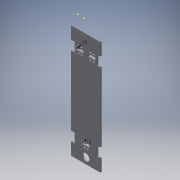
# Autodesk Inventor part: XCartFloor
Saved by Autodesk Inventor 2019 (Build 230136000, 136)
## iProperties
Created: 2019-08-19
Part Number: XCartFloor
Material: Generic
Document SubType Name: Modeling
Designer: Bruno
Density: 1 g/cm^3
Appearance: Default
Author: Bruno
Autodesk Inventor part; units mm, degrees
ref_plane "YZ Plane" through (0, 0, 0) normal (1, 0, 0) x (0, 1, 0)
ref_plane "XZ Plane" through (0, 0, 0) normal (0, 1, 0) x (-1, 0, 0)
ref_plane "XY Plane" through (0, 0, 0) normal (0, 0, 1) x (1, 0, 0)
sketch "Sketch1" plane through (0, 0, 0) normal (0, 0, 1) x (1, 0, 0)
  line L0 (100.0979, -38.5222) -> (0.0979, -38.5222)
  line L1 (0.0979, -426.5222) -> (100.0979, -426.5222)
  line L2 (82.7645, -93.1222) -> (58.7645, -93.1222)
  line L3 (58.7645, -93.1222) -> (58.7645, -101.9222)
  line L4 (58.7645, -101.9222) -> (82.7645, -101.9222)
  line L5 (82.7645, -101.9222) -> (82.7645, -93.1222)
  line L6 (41.4312, -93.1222) -> (17.4312, -93.1222)
  line L7 (17.4312, -93.1222) -> (17.4312, -101.9222)
  line L8 (17.4312, -101.9222) -> (41.4312, -101.9222)
  line L9 (41.4312, -101.9222) -> (41.4312, -93.1222)
  line L10 (38.0979, -363.1222) -> (62.0979, -363.1222)
  line L11 (62.0979, -363.1222) -> (62.0979, -371.9222)
  line L12 (62.0979, -371.9222) -> (38.0979, -371.9222)
  line L13 (38.0979, -371.9222) -> (38.0979, -363.1222)
  line L14 (173.8639, -93.5222) -> (-221.1361, -93.5222)
  line L15 (173.8639, -101.5222) -> (-221.1361, -101.5222)
  line L16 (173.8639, -371.5222) -> (-221.1361, -371.5222)
  line L17 (173.8639, -363.5222) -> (-221.1361, -363.5222)
  line L18 (34.8712, -93.1222) -> (34.8712, -93.5222) construction
  line L19 (34.8712, -101.5222) -> (34.8712, -101.9222) construction
  line L20 (58.7645, -93.1222) -> (41.4312, -93.1222) construction
  line L21 (10.9151, -363.1222) -> (10.9151, -363.5222) construction
  line L22 (10.9151, -371.5222) -> (10.9151, -371.9222) construction
  line L23 (38.0979, -363.1222) -> (12.0979, -363.1222) construction
  line L24 (62.0979, -363.1222) -> (88.0979, -363.1222) construction
  line L25 (0, 0) -> (0, -9.7735) construction
  circle A0 centre (65.5981, -390.5222) radius 1.625
  circle A1 centre (65.5981, -421.5222) radius 1.625
  circle A2 centre (34.5981, -421.5222) radius 1.625
  circle A3 centre (34.5981, -390.5222) radius 1.625
  line L26 (65.5981, -390.5222) -> (34.5981, -390.5222) construction
  line L27 (34.5981, -390.5222) -> (34.5981, -421.5222) construction
  line L28 (34.5981, -421.5222) -> (65.5981, -421.5222) construction
  line L29 (65.5981, -421.5222) -> (65.5981, -390.5222) construction
  line L30 (34.5981, -390.5222) -> (0.0979, -390.3972) construction
  line L31 (65.5981, -390.5222) -> (100.0979, -390.7595) construction
  circle A4 centre (50.0981, -406.0222) radius 12.5
  line L32 (50.0981, -390.5222) -> (50.0981, -406.0222) construction
  line L33 (50.0981, -406.0222) -> (65.5981, -406.0222) construction
  line L34 (72.2645, -84.1222) -> (80.2645, -84.1222)
  line L35 (80.2645, -84.1222) -> (80.2645, -88.1222)
  line L36 (80.2645, -88.1222) -> (72.2645, -88.1222)
  line L37 (72.2645, -88.1222) -> (72.2645, -84.1222)
  line L38 (80.2645, -88.1222) -> (82.7645, -88.1222) construction
  line L39 (82.7645, -88.1222) -> (82.7645, -93.1222) construction
  line L40 (69.2645, -84.1222) -> (61.2645, -84.1222)
  line L41 (61.2645, -84.1222) -> (61.2645, -88.1222)
  line L42 (61.2645, -88.1222) -> (69.2645, -88.1222)
  line L43 (69.2645, -88.1222) -> (69.2645, -84.1222)
  line L44 (58.7645, -93.1222) -> (58.7645, -88.1222) construction
  line L45 (58.7645, -88.1222) -> (61.2645, -88.1222) construction
  line L46 (72.2645, -106.9222) -> (80.2645, -106.9222)
  line L47 (80.2645, -106.9222) -> (80.2645, -110.9222)
  line L48 (80.2645, -110.9222) -> (72.2645, -110.9222)
  line L49 (72.2645, -110.9222) -> (72.2645, -106.9222)
  line L50 (80.2645, -106.9222) -> (80.2645, -101.9222) construction
  line L51 (69.2645, -106.9222) -> (61.2645, -106.9222)
  line L52 (61.2645, -106.9222) -> (61.2645, -110.9222)
  line L53 (61.2645, -110.9222) -> (69.2645, -110.9222)
  line L54 (69.2645, -110.9222) -> (69.2645, -106.9222)
  line L55 (38.9312, -84.1222) -> (30.9312, -84.1222)
  line L56 (30.9312, -84.1222) -> (30.9312, -88.1222)
  line L57 (30.9312, -88.1222) -> (38.9312, -88.1222)
  line L58 (38.9312, -88.1222) -> (38.9312, -84.1222)
  line L59 (27.9312, -84.1222) -> (19.9312, -84.1222)
  line L60 (19.9312, -84.1222) -> (19.9312, -88.1222)
  line L61 (19.9312, -88.1222) -> (27.9312, -88.1222)
  line L62 (27.9312, -88.1222) -> (27.9312, -84.1222)
  line L63 (30.9312, -106.9222) -> (38.9312, -106.9222)
  line L64 (38.9312, -106.9222) -> (38.9312, -110.9222)
  line L65 (38.9312, -110.9222) -> (30.9312, -110.9222)
  line L66 (30.9312, -110.9222) -> (30.9312, -106.9222)
  line L67 (27.9312, -106.9222) -> (19.9312, -106.9222)
  line L68 (19.9312, -106.9222) -> (19.9312, -110.9222)
  line L69 (19.9312, -110.9222) -> (27.9312, -110.9222)
  line L70 (27.9312, -110.9222) -> (27.9312, -106.9222)
  line L71 (41.4312, -93.1222) -> (41.4312, -88.1222) construction
  line L72 (41.4312, -88.1222) -> (38.9312, -88.1222) construction
  line L73 (17.4312, -93.1222) -> (17.4312, -88.1222) construction
  line L74 (17.4312, -88.1222) -> (19.9312, -88.1222) construction
  line L75 (51.5979, -354.1222) -> (59.5979, -354.1222)
  line L76 (59.5979, -354.1222) -> (59.5979, -358.1222)
  line L77 (59.5979, -358.1222) -> (51.5979, -358.1222)
  line L78 (51.5979, -358.1222) -> (51.5979, -354.1222)
  line L79 (48.5979, -354.1222) -> (40.5979, -354.1222)
  line L80 (40.5979, -354.1222) -> (40.5979, -358.1222)
  line L81 (40.5979, -358.1222) -> (48.5979, -358.1222)
  line L82 (48.5979, -358.1222) -> (48.5979, -354.1222)
  line L83 (51.5979, -376.9222) -> (59.5979, -376.9222)
  line L84 (59.5979, -376.9222) -> (59.5979, -380.9222)
  line L85 (59.5979, -380.9222) -> (51.5979, -380.9222)
  line L86 (51.5979, -380.9222) -> (51.5979, -376.9222)
  line L87 (48.5979, -376.9222) -> (40.5979, -376.9222)
  line L88 (40.5979, -376.9222) -> (40.5979, -380.9222)
  line L89 (40.5979, -380.9222) -> (48.5979, -380.9222)
  line L90 (48.5979, -380.9222) -> (48.5979, -376.9222)
  line L91 (59.5979, -358.1222) -> (62.0979, -358.1222) construction
  line L92 (62.0979, -358.1222) -> (62.0979, -363.1222) construction
  line L93 (38.0979, -363.1222) -> (38.0979, -358.1222) construction
  line L94 (38.0979, -358.1222) -> (40.5979, -358.1222) construction
  line L95 (59.5979, -376.9222) -> (59.5979, -371.9222) construction
  circle A5 centre (73.5, -50.5222) radius 2.125
  circle A6 centre (26.5, -50.5222) radius 2.125
  line L96 (73.5, -50.5222) -> (100, -50.5222) construction
  line L97 (26.5, -50.5222) -> (0, -50.5222) construction
  line L98 (96.5, -57.5222) -> (88.5, -57.5222) projected
  line L99 (11.5, -57.5222) -> (3.5, -57.5222) projected
  line L100 (8, -43.5222) -> (8, -57.5222) projected
  line L101 (7, -57.5222) -> (7, -43.5222) projected
  line L102 (93, -43.5222) -> (93, -57.5222) projected
  line L103 (92, -57.5222) -> (92, -43.5222) projected
  line L104 (7.5, -57.5222) -> (7.5, -426.5222) construction
  line L105 (92.5, -57.5222) -> (92.5, -426.5222) construction
  circle A7 centre (92.5, -419.5222) radius 2.125
  circle A8 centre (92.5, -392.5222) radius 2.125
  circle A9 centre (7.5, -419.5222) radius 2.125
  circle A10 centre (7.5, -392.5222) radius 2.125
  line L106 (92.5, -419.5222) -> (7.5, -419.5222) construction
  line L107 (92.5, -392.5222) -> (7.5, -392.5222) construction
  line L108 (100.0979, -38.5222) -> (100.0979, -81.5222)
  line L109 (100.0979, -81.5222) -> (88.0979, -81.5222)
  line L110 (88.0979, -81.5222) -> (88.0979, -113.5222)
  line L111 (88.0979, -113.5222) -> (100.0979, -113.5222)
  line L112 (100.0979, -351.5222) -> (88.0979, -351.5222)
  line L113 (88.0979, -351.5222) -> (88.0979, -383.5222)
  line L114 (88.0979, -383.5222) -> (100.0979, -383.5222)
  line L115 (100.0979, -383.5222) -> (100.0979, -426.5222)
  line L116 (100.0979, -81.5222) -> (100.0979, -93.5222) construction
  line L117 (100.0979, -101.5222) -> (100.0979, -113.5222) construction
  line L118 (0.0979, -38.5222) -> (0.0979, -81.5222)
  line L119 (0.0979, -81.5222) -> (12.0979, -81.5222)
  line L120 (12.0979, -81.5222) -> (12.0979, -113.5222)
  line L121 (12.0979, -113.5222) -> (0.0979, -113.5222)
  line L122 (0.0979, -351.5222) -> (12.0979, -351.5222)
  line L123 (12.0979, -351.5222) -> (12.0979, -383.5222)
  line L124 (12.0979, -383.5222) -> (0.0979, -383.5222)
  line L125 (0.0979, -383.5222) -> (0.0979, -426.5222)
  line L126 (98.1469, -351.5222) -> (98.1469, -363.5222) construction
  line L127 (98.1469, -383.5222) -> (98.1469, -371.5222) construction
  line L128 (17.4312, -93.1222) -> (12.0979, -93.1222) construction
  line L129 (82.7645, -93.1222) -> (88.0979, -93.1222) construction
  line L130 (82.7645, -97.5222) -> (100.0979, -97.5222) construction
  line L131 (58.7645, -97.5222) -> (41.4312, -97.5222) construction
  line L132 (17.4312, -97.5222) -> (0.0979, -97.5222) construction
  line L133 (38.0979, -367.5222) -> (0.0979, -367.5222) construction
  line L134 (62.0979, -367.5222) -> (100.0979, -367.5222) construction
  line L135 (100.0979, -113.5222) -> (100.0979, -207.5222)
  line L136 (100.0979, -207.5222) -> (88.0979, -207.5222)
  line L137 (88.0979, -207.5222) -> (88.0979, -257.5222)
  line L138 (88.0979, -257.5222) -> (100.0979, -257.5222)
  line L139 (100.0979, -257.5222) -> (100.0979, -351.5222)
  line L140 (0.0979, -113.5222) -> (0.0979, -207.5222)
  line L141 (0.0979, -207.5222) -> (12.0979, -207.5222)
  line L142 (12.0979, -207.5222) -> (12.0979, -257.5222)
  line L143 (12.0979, -257.5222) -> (0.0979, -257.5222)
  line L144 (0.0979, -257.5222) -> (0.0979, -351.5222)
  dimension "d1" = 24
  dimension "d2" = 8.8
  dimension "d3" = 100
  dimension "d9" = 55
  dimension "d10" = 55
  dimension "d11" = 3.25
  dimension "d12" = 31
  dimension "d13" = 5
  dimension "d14" = 25
  dimension "d15" = 4
  dimension "d16" = 8
  dimension "d17" = 5
  dimension "d18" = 2.5
  dimension "d19" = 4.25
  dimension "d20" = 4.25
  dimension "d21" = 47
  dimension "d22" = 12
  dimension "d23" = 4.25
  dimension "d24" = 4.25
  dimension "d25" = 27
  dimension "d26" = 7
  dimension "d27" = 4.25
  dimension "d28" = 4.25
  dimension "d29" = 32
  dimension "d30" = 12
  dimension "d31" = 50
  constraints: 278 end point, 62 point on line, 46 equal length, 46 perpendicular, 34 parallel, 28 horizontal, 18 collinear, 15 vertical, 11 centre point, 10 midpoint, 3 equal radius, 8 other
  measures "d1" distance of L3.end L4.end
  measures "d2" distance of L2.end L3.end
  measures "d3" distance of L0.start L0.end
  measures "d9" distance between parallel lines of L0 L14
  measures "d10" distance between parallel lines of L1 L16
  measures "d11" diameter of A0
  measures "d12" distance of L28.end L26.start
  measures "d13" distance between parallel lines of L1 L28
  measures "d14" diameter of A4
  measures "d15" distance of L34.end L35.end
  measures "d16" distance of L34.start L34.end
  measures "d17" distance of L38.end L2.start
  measures "d18" distance of L35.end L38.end
  measures "d19" diameter of A5
  measures "d20" diameter of A6
  measures "d21" distance of L97.start L96.start
  measures "d22" distance between parallel lines of L0 L96
  measures "d23" diameter of A7
  measures "d24" diameter of A8
  measures "d25" distance of L106.start L107.start
  measures "d26" distance from line of L1 L106.start
  measures "d27" diameter of A9
  measures "d28" diameter of A10
  measures "d29" distance of L109.end L110.end
  measures "d30" distance of L110.end L111.end
  measures "d31" distance of L136.end L137.end
extrude "Extrusion1" add sketch "Sketch1" along normal blind 5 contours L108 L109 L110 L14 L5 L2 L3 L9 L6 L7 L120 L119 L118 L0 | L110 L15 L5 L14 | L14 L7 L15 L120 | L110 L111 L135 L136 L137 L138 L139 L112 L113 L17 L11 L10 L13 L123 L122 L144 L143 L142 L141 L140 L121 L120 L15 L7 L8 L9 L3 L4 L5 | L3 L15 L9 L14 | L113 L16 L11 L17 | L17 L13 L16 L123 | L113 L114 L115 L1 L125 L124 L123 L16 L13 L12 L11
sketch "Sketch2" plane through (17.4312, -101.9222, 0) normal (1, 0, 0) x (0, 0, -1)
  circle A0 centre (6.0737, 4.4) radius 7.5
  point P0 (0, 101.9222)
  point P1 (0, 8.8)
  point P2 (0, 0)
  dimension "d6" = 15
  constraints: 2 point on circle, 1 centre point
  measures "d6" diameter of A0
sketch "Sketch3" plane through (38.0979, -371.9222, 0) normal (1, 0, 0) x (0, 0, -1)
  circle A0 centre (6.0737, 4.4) radius 7.5
  point P0 (0, 371.9222)
  point P1 (0, 8.8)
  point P2 (0, 0)
  dimension "d8" = 15
  constraints: 2 point on circle, 1 centre point
  measures "d8" diameter of A0
body "Solid1"
